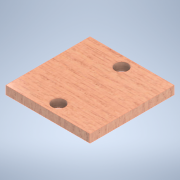
# Autodesk Inventor part: Ba
Saved by Autodesk Inventor 2021 (Build 250183000, 183)
## iProperties
Created: 2021-07-06
Part Number: Ba
Material: Wood (Oak)
Document SubType Name: Modeling
Designer: KAVYA
Density: 0.76 g/cm^3
Appearance: White Oak - Natural Medium Gloss
Author: KAVYA
Autodesk Inventor part; units mm, degrees
ref_plane "YZ Plane" through (0, 0, 0) normal (1, 0, 0) x (0, 1, 0)
ref_plane "XZ Plane" through (0, 0, 0) normal (0, 1, 0) x (-1, 0, 0)
ref_plane "XY Plane" through (0, 0, 0) normal (0, 0, 1) x (1, 0, 0)
sketch "Sketch1" plane through (0, 0, 0) normal (0, 1, 0) x (-1, 0, 0)
  line L0 (0, 0) -> (-100, 0)
  line L1 (-100, 0) -> (-100, -100)
  line L2 (-100, -100) -> (0, -100)
  line L3 (0, -100) -> (0, 0)
  dimension "d0" = 100
  dimension "d1" = 100
  constraints: 8 end point, 2 parallel, 1 horizontal, 1 perpendicular
  measures "d0" distance of L2.end L1.end
  measures "d1" distance of L1.end L0.end
extrude "Extrusion1" add sketch "Sketch1" along normal blind 10
sketch "Sketch2" plane through (0, 10, 0) normal (0, 1, 0) x (1, 0, 0)
  circle A0 centre (50, 12.5) radius 7.75
  circle A1 centre (50, 87.5) radius 7.75
  line L0 (0, 0) -> (100, 0) projected
  line L1 (0, 100) -> (0, 0) projected
  line L2 (100, 100) -> (0, 100) projected
  dimension "d4" = 15.5
  dimension "d5" = 15.5
  dimension "d6" = 12.5
  dimension "d7" = 50
  dimension "d8" = 12.5
  dimension "d9" = 50
  constraints: 2 centre point
  measures "d4" diameter of A0
  measures "d5" diameter of A1
  measures "d6" distance from line of L0 A0.centre
  measures "d7" distance from line of L1 A0.centre
  measures "d8" distance from line of L2 A1.centre
  measures "d9" distance from line of L1 A1.centre
extrude "Extrusion2" cut sketch "Sketch2" against normal blind 10
body "Solid1"
